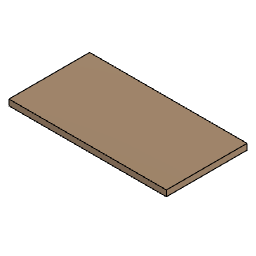
Connection box lid (Autodesk Fusion 360 design; units mm, degrees)
Autodesk Fusion 360 part; units mm, degrees
sketch "Sketch1" plane through (0, 0, 0) normal (0, 0, 1) x (1, 0, 0)
  line L0 (74, -35) -> (-74, -35)
  line L1 (-74, -35) -> (-74, 35)
  line L2 (-74, 35) -> (74, 35)
  line L3 (74, 35) -> (74, -35)
  line L4 (74, -35) -> (-74, 35) construction
  line L5 (-74, -35) -> (74, 35) construction
  line L6 (80, 41) -> (-80, 41)
  line L7 (-80, 41) -> (-80, -41)
  line L8 (-80, -41) -> (80, -41)
  line L9 (80, -41) -> (80, 41)
  line L10 (80, 41) -> (-80, -41) construction
  line L11 (-80, 41) -> (80, -41) construction
  dimension "d1" = 148
  dimension "d2" = 70
  dimension "d3" = 160
  dimension "d4" = 82
  constraint perpendicular L0 L1
  constraint parallel L0 L2
  constraint parallel L1 L3
  constraint horizontal L0
  constraint coincident L4 origin
  constraint coincident L5 origin
  constraint perpendicular L6 L7
  constraint parallel L6 L8
  constraint parallel L7 L9
  constraint horizontal L6
  constraint coincident L10 origin
  constraint coincident L11 origin
  measures "d1" distance of L1.end L2.end
  measures "d2" distance of L0.end L1.end
  measures "d3" distance of L7.end L8.end
  measures "d4" distance of L6.end L7.end
extrude "Extrude1" add sketch "Sketch1" against normal blind 6 contours L0 L1 L2 L3 makes body 1
extrude "Extrude2" add sketch "Sketch1" along normal blind 6 separate body contours L0 L1 L2 L3 | L6 L7 L8 L9 makes body 2
equation "d3 = d1 + 12 mm"
equation "d4 = d2 + 12 mm"
named bodies: "Inset", "Lid"
